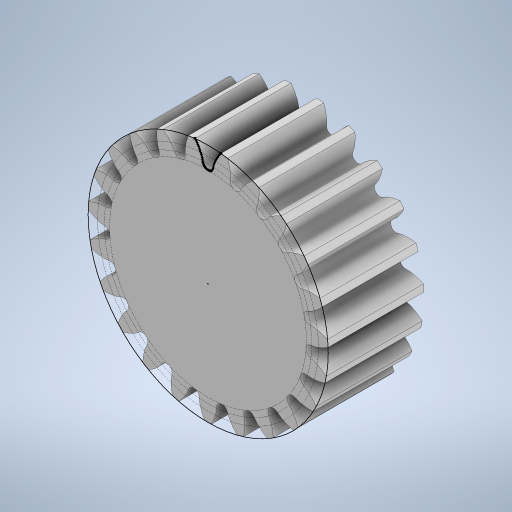
# Autodesk Inventor part: Gear
Saved by Autodesk Inventor 2023.2 (Build 272271000, 271)
## iProperties
Created: 2023-10-07
Part Number: Gear
Material: Generic
Document SubType Name: Modeling
Designer: 271663e
Density: 1 g/cm^3
Appearance: Default
Author: 271663e
Autodesk Inventor part; units mm, degrees
ref_plane "YZ Plane" through (0, 0, 0) normal (1, 0, 0) x (0, 1, 0)
ref_plane "XZ Plane" through (0, 0, 0) normal (0, 1, 0) x (-1, 0, 0)
ref_plane "XY Plane" through (0, 0, 0) normal (0, 0, 1) x (1, 0, 0)
sketch "Sketch1" plane through (0, 0, 0) normal (0, 0, 1) x (1, 0, 0)
  spline S0 degree 3 poles (-2.6985, 24.8539) (-2.6322, 24.7627) (-2.4996, 24.5802) (-2.311, 24.2992) (-2.1302, 24.0131) (-1.9587, 23.7214) (-1.7971, 23.424) (-1.6466, 23.1209) (-1.5085, 22.8119) (-1.3842, 22.497) (-1.2776, 22.1759) (-1.1883, 21.8489) (-1.1509, 21.569) (-1.0996, 21.3491) (-1.0454, 21.1886) (-0.9752, 21.0345) (-0.8879, 20.8889) (-0.7953, 20.782) (-0.7134, 20.7043) (-0.6452, 20.6541) (-0.5743, 20.6075) (-0.4977, 20.5715) (-0.4194, 20.539) (-0.3371, 20.5189) (-0.2539, 20.5028) (-0.1409, 20.4983) (0, 20.5011) (0.1409, 20.4983) (0.2539, 20.5028) (0.3371, 20.5189) (0.4194, 20.539) (0.4977, 20.5715) (0.5743, 20.6075) (0.6452, 20.6541) (0.7134, 20.7043) (0.7953, 20.782) (0.8879, 20.8889) (0.9752, 21.0345) (1.0454, 21.1886) (1.0996, 21.3491) (1.1509, 21.569) (1.1883, 21.8489) (1.2776, 22.1759) (1.3842, 22.497) (1.5085, 22.8119) (1.6466, 23.1209) (1.7971, 23.424) (1.9587, 23.7214) (2.1302, 24.0131) (2.311, 24.2992) (2.4996, 24.5802) (2.6322, 24.7627) (2.6985, 24.8539) knots 0 0 0 0 0.033836 0.067673 0.101509 0.135345 0.169181 0.203016 0.236851 0.270686 0.304518 0.338347 0.372179 0.389096 0.40601 0.422918 0.439825 0.456722 0.465184 0.473643 0.482101 0.490559 0.499017 0.507474 0.515933 0.52439 0.541308 0.558227 0.566684 0.575142 0.5836 0.592057 0.600515 0.608974 0.617432 0.625894 0.642791 0.659698 0.676606 0.693521 0.710438 0.744269 0.778098 0.811931 0.845765 0.8796 0.913435 0.947271 0.981107 1.014944 1.04878 1.082616 1.082616 1.082616 1.082616
  circle A0 centre (0, 0) radius 20.5 construction
  circle A1 centre (0, 0) radius 21.6129 construction
  circle A2 centre (0, 0) radius 23 construction
  circle A3 centre (0, 0) radius 25
  point P0 (-2.5013, 24.579)
  point P1 (-2.3123, 24.2983)
  point P2 (-2.1317, 24.0122)
  point P3 (-1.9603, 23.7204)
  point P4 (-1.799, 23.423)
  point P5 (-1.6487, 23.1199)
  point P6 (-1.5108, 22.8109)
  point P7 (-1.3871, 22.496)
  point P8 (-1.2804, 22.1749)
  point P9 (-1.1957, 21.8474)
  point P10 (-1.1363, 21.5144)
  point P11 (-1.097, 21.3498)
  point P12 (-1.0427, 21.1896)
  point P13 (-0.9723, 21.0359)
  point P14 (-0.8839, 20.8918)
  point P15 (-0.7742, 20.7633)
  point P16 (-0.7123, 20.7056)
  point P17 (-0.6447, 20.6547)
  point P18 (-0.5734, 20.6093)
  point P19 (-0.4974, 20.5721)
  point P20 (-0.4187, 20.5411)
  point P21 (-0.3369, 20.5196)
  point P22 (-0.2536, 20.5049)
  point P23 (-0.1692, 20.5)
  point P24 (0, 20.5)
  point P25 (0.1692, 20.5)
  point P26 (0.2536, 20.5049)
  point P27 (0.3369, 20.5196)
  point P28 (0.4187, 20.5411)
  point P29 (0.4974, 20.5721)
  point P30 (0.5734, 20.6093)
  point P31 (0.6447, 20.6547)
  point P32 (0.7123, 20.7056)
  point P33 (0.7742, 20.7633)
  point P34 (0.8839, 20.8918)
  point P35 (0.9723, 21.0359)
  point P36 (1.0427, 21.1896)
  point P37 (1.097, 21.3498)
  point P38 (1.1363, 21.5144)
  point P39 (1.1957, 21.8474)
  point P40 (1.2804, 22.1749)
  point P41 (1.3871, 22.496)
  point P42 (1.5108, 22.8109)
  point P43 (1.6487, 23.1199)
  point P44 (1.799, 23.423)
  point P45 (1.9603, 23.7204)
  point P46 (2.1317, 24.0122)
  point P47 (2.3123, 24.2983)
  point P48 (2.5013, 24.579)
  constraints: 4 centre point, 2 point on circle, 107 other
extrude "Extrusion1" add sketch "Sketch1" against normal blind 20
extrude "Extrusion2" cut sketch "Sketch1" against normal blind 20 contours A3 S0 picked at (-0.3308, 23.8142)
pattern_circular "Circular Pattern1" count 23 over 360 about axis through (0, 0, 0) along (0, 0, -1) of "Extrusion2"
equation "\"d0\" = FaceWidth"
equation "\"Module\" = 2"
equation "\"PressureAngle\" = 20deg"
equation "\"UnitProfileClearance\" = 0.25"
equation "\"UnitRoundRadius\" = 0.35"
equation "\"RootDiameter\" = 41"
equation "\"BaseDiameter\" = 43.22586"
equation "\"PitchDiameter\" = 46"
equation "\"FaceWidth\" = 20"
equation "\"HelixAngle\" = 0"
equation "\"UnitCorrection\" = 0"
equation "\"UnitAddendumModification\" = 0"
equation "\"CircularPitch\" = 6.283185"
equation "\"UnitBacklashShift\" = 0"
equation "\"TotalToolShift\" = 0"
equation "\"IsInternal\" = 0"
body "Solid1"
